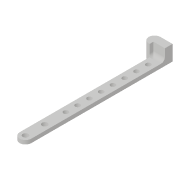
# Autodesk Inventor part: CollectorArmRear4_623long
Saved by Autodesk Inventor 2018 (Build 220112000, 112)
## iProperties
Created: 2019-02-19
Part Number: CollectorArmRear4_623long
Material: Generic
Document SubType Name: Modeling
Designer: ball
Density: 1 g/cm^3
Appearance: Default
Author: ball
Autodesk Inventor part; units mm, degrees
ref_plane "YZ Plane" through (0, 0, 0) normal (1, 0, 0) x (0, 1, 0)
ref_plane "XZ Plane" through (0, 0, 0) normal (0, 1, 0) x (-1, 0, 0)
ref_plane "XY Plane" through (0, 0, 0) normal (0, 0, 1) x (1, 0, 0)
sketch "Sketch1" plane through (0, 0, 0) normal (0, 1, 0) x (-1, 0, 0)
  line L0 (0, 0) -> (10.16, 0)
  line L1 (9.525, 9.6012) -> (9.525, 117.4242)
  line L2 (0, 117.4242) -> (0, 0)
  circle A0 centre (4.7625, 117.4242) radius 2.2479
  circle A1 centre (4.7625, 101.4222) radius 2.2479
  circle A2 centre (4.7625, 83.8708) radius 1.9685
  arc A3 (10.16, 0) -> (10.16, 9.6012) centre (10.16, 4.8006) ccw
  line L3 (10.16, 9.6012) -> (9.525, 9.6012)
  circle A4 centre (4.7625, 74.0918) radius 1.9685
  circle A5 centre (4.7625, 64.3128) radius 1.9685
  circle A6 centre (4.7625, 54.5338) radius 1.9685
  circle A7 centre (4.7625, 44.7548) radius 1.9685
  circle A8 centre (4.7625, 34.9758) radius 1.9685
  circle A9 centre (4.7625, 25.1968) radius 1.9685
  circle A10 centre (4.7625, 15.4178) radius 1.9685
  arc A11 (9.525, 117.4242) -> (0, 117.4242) centre (4.7625, 117.4747) ccw
  dimension "d0" = 9.525
  dimension "d4" = 4.4958
  dimension "d5" = 4.4958
  dimension "d6" = 16.002
  dimension "d7" = 3.937
  dimension "d8" = 17.5514
  dimension "d16" = 4.8006
  dimension "d17" = 10.16
  dimension "d18" = 117.4242
  dimension "d21" = 9.779
  dimension "d27" = 4.7628
  dimension "d28" = 0
  dimension "d29" = 0
  constraints: 12 centre point, 8 end point, 4 point on circle, 2 perpendicular, 1 coincident, 1 horizontal, 1 parallel, 1 vertical, 14 other
  measures "d0" distance of L2.start L1.end
  measures "d4" diameter of A0
  measures "d5" diameter of A1
  measures "d6" distance of A1.centre A0.centre
  measures "d7" diameter of A2
  measures "d8" distance of A2.centre A1.centre
  measures "d16" distance from line of L0 point (10.16, 4.801)
  measures "d17" distance from line of L2 point (10.16, 4.801)
  measures "d18" distance from line of L0 A0.centre
  measures "d21" distance of A2.centre A4.centre
  measures "d27" radius of A11
  measures "d28" vertical distance of L1.end A0.centre
  measures "d29" vertical distance of L2.start A0.centre
extrude "Extrusion1" add sketch "Sketch1" along normal blind 3.175
sketch "Sketch2" plane through (0, 3.175, 0) normal (0, 1, 0) x (1, 0, 0)
  line L0 (-9.525, -9.6012) -> (-9.525, -6.35)
  line L1 (-9.525, -6.35) -> (0, -6.35)
  line L2 (0, -117.4242) -> (0, 0) projected
  line L3 (0, -6.35) -> (0, 0)
  arc A0 (-10.16, 0) -> (-10.16, -9.6012) centre (-10.16, -4.8006) ccw projected
  arc A1 (-10.16, 0) -> (-10.239, -9.6012) centre (-10.1597, -4.8009) ccw
  line L4 (-10.16, -9.6012) -> (-9.525, -9.6012) projected
  line L5 (-9.525, -9.6012) -> (-10.16, -9.6012)
  line L6 (0, 0) -> (-10.16, 0) projected
  line L7 (-10.16, 0) -> (0, 0)
  constraints: 10 end point, 3 point on circle, 2 perpendicular, 1 centre point, 1 collinear, 1 horizontal, 1 vertical
extrude "Extrusion2" add sketch "Sketch2" along normal blind 9.525
fillet "Fillet1" radius 3.175 2 edges at (-4.7625, 3.175, 6.35) (-9.525, 3.175, 7.9756)
body "Solid1"
